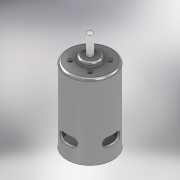
# Autodesk Inventor part: dc_motor
Saved by Autodesk Inventor 2020 (Build 240168000, 168)
## iProperties
Created: 2020-06-18
Part Number: dc_motor
Material: Generic
Document SubType Name: Modeling
Designer: pc-konvi
Density: 1 g/cm^3
Appearance: Default
Author: pc-konvi
Autodesk Inventor part; units mm, degrees
ref_plane "YZ Plane" through (0, 0, 0) normal (1, 0, 0) x (0, 1, 0)
ref_plane "XZ Plane" through (0, 0, 0) normal (0, 1, 0) x (-1, 0, 0)
ref_plane "XY Plane" through (0, 0, 0) normal (0, 0, 1) x (1, 0, 0)
sketch "Sketch1" plane through (0, 0, 0) normal (0, 1, 0) x (-1, 0, 0)
  circle A0 centre (0, 0) radius 25.9
  circle A1 centre (0, 0) radius 16 construction
  line L0 (0, 0) -> (11.3137, -11.3137) construction
  line L1 (0, 0) -> (16, 0) construction
  circle A2 centre (11.3137, -11.3137) radius 2.5
  circle A3 centre (0, 0) radius 10.85
  dimension "d1" = 32
  dimension "d0" = 51.8
  dimension "d2" = 45
  dimension "d3" = 5
  dimension "d11" = 21.7
  dimension "d28" = 11.3137
  constraints: 4 coincident, 4 end point, 3 centre point, 1 equal length, 1 horizontal, 3 other
  measures "d0" diameter of A0
  measures "d2" angle of L0 L1
  measures "d3" diameter of A2
  measures "d11" diameter of A3
  measures "d28" horizontal distance of point (0, 0) L0.end
extrude "Extrusion1" add sketch "Sketch1" against normal blind 85 contours A0 | A2 | A3
extrude "Extrusion2" cut sketch "Sketch1" against normal blind 10 contours A2
pattern_circular "Circular Pattern1" count 4 over 360 about axis through (0, -10, 0) along (0, 1, 0) of "Extrusion2"
extrude "Extrusion3" add sketch "Sketch1" along normal blind 5.5 contours A3
sketch "Sketch2" plane through (0, 5.5, 0) normal (0, 1, 0) x (1, 0, 0)
  circle A0 centre (0, 0) radius 3.175
  dimension "d14" = 6.35
  constraints: 1 centre point, 1 coincident
  measures "d14" diameter of A0
extrude "Extrusion4" add sketch "Sketch2" along normal blind 21.5
fillet "Fillet1" radius 2.5 2 edges at (10.85, 5.5, 0) (25.9, 0, 0)
sketch "Sketch3" plane through (0, 0, 0) normal (1, 0, 0) x (0, 1, 0)
  line L0 (-70, 10) -> (-60, 10)
  line L1 (-60, 10) -> (-60, -10)
  line L2 (-60, -10) -> (-70, -10)
  line L3 (-70, -10) -> (-70, 10)
  line L4 (0, 10.85) -> (0, -10.85) projected
  circle A0 centre (-65, 5) radius 5
  circle A1 centre (-65, -5) radius 5
  point P0 (0, 0)
  point P1 (-60, 0)
  point P2 (-70, -5)
  point P3 (-60, -5)
  point P4 (-60, 5)
  point P5 (-70, 5)
  dimension "d19" = 60
  dimension "d20" = 70
  dimension "d21" = 20
  constraints: 8 end point, 4 tangent, 2 centre point, 2 parallel, 1 horizontal, 1 horizontal alignment, 1 midpoint, 1 perpendicular
  measures "d19" distance between parallel lines of L4 L1
  measures "d20" distance between parallel lines of L4 L3
  measures "d21" distance of L2.end L0.start
shell "Shell1" thickness 2.5 removed faces 4 at (-11.7147, -6.6667, 13.7813) at (10.5758, -10, 11.701) at (11.701, -10, -10.5758) at (-10.5758, -10, -11.701)
extrude "Extrusion5" cut sketch "Sketch3" along normal mid plane 85 contours A0 | A0 A1 L3 | L1 A1 A0 | A1
pattern_circular "Circular Pattern2" count 4 over 360 about axis through (0, -10, 0) along (0, 1, 0) of "Extrusion5"
body "Solid1"
